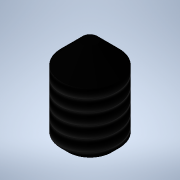
# Autodesk Inventor part: 623890036_2
Saved by Autodesk Inventor 2021 (Build 250183000, 183)
## iProperties
Created: 2026-04-17
Part Number: 623890036_2
Material: Generic
Catalog Web Link: www.3dfindit.com
Description: gst_din_4027-Grub screw, Adjusting Rings (Shaft Collars with Set Screw)  DIN 705 A
Vendor: MAEDLER
Document SubType Name: Modeling
Designer: psAdmin
Manufacturer: MAEDLER
Mass: 0.00736438 g
Surface Area: 0.231524 cm^2
Volume: 0.00736438 cm^3
Density: 1 g/cm^3
Appearance: PSOLRGB-44-44-44
Category: PARTsolutions
Company: MAEDLER
Title: 623890036
Author: Cadenas PARTsolutions
Comments: Grub screw, Adjusting Rings (Shaft Collars with Set Screw)  DIN 705 A
PSOL_IDENT_0: {$CADENAS_DATA/23d-libs/maedler/antriebselemente/klemmringe_stellringe/stellringe/din705a/din_705a_i
PSOL_IDENT_1: s_4027/gst_din_4027.prj},168 {VTYP=3D},{NB=623890036_2},{LINA=623890036},{NN=gst_din_4027},{DATE=01.
PSOL_IDENT_2: 12.2025 10:57:12},{GEOMDATE=20.02.2024 10:31:27},{VERSION=},{LINEID=2570},{WBVAR=},{WBNUMERIC=}  {NB=
PSOL_IDENT_3: 623890036_2},{LINA=623890036},{KT=DUMMY},{ARTNR=623890036},{WEBSHOP=Produktdetails / Katalogseite /
PSOL_IDENT_4: Montageanleitung},{MATK=Stahl brüniert},{MAT=Stahl brüniert, Gewindestift mit Festigkeit 45H oder 12
PSOL_IDENT_5: .9, schwarz},{AUSF=mit 1x Gewindestift mit Innensechskant DIN EN ISO 4027},{D1=3},{D2=7},{B=5},{SCHR=
PSOL_IDENT_6: M2 x 3},{GEW=0.123},{D3=1.570},{SCHRAUBE=2.0},{DD1=0.00},{N=0.0},{T=0.0},{DDD1=0.5},{SW=0.9},{T1=0.8
PSOL_IDENT_7: },{SCHRL=3},{SCHRUEB=1.0},{TYP=2},{CTN=73182900}
NB: 623890036_2
NN: gst_din_4027
NT: Grub screw, Adjusting Rings (Shaft Collars with Set Screw)  DIN 705 A
NBSYN: $ARTNR._2
LINA: 623890036
CATALOG: MÄDLER
ARTNR: 623890036
WEBSHOP: Produktdetails / Katalogseite / Montageanleitung
MATK: Stahl brüniert
MAT: Stahl brüniert, Gewindestift mit Festigkeit 45H oder 12.9, schwarz
AUSF: mit 1x Gewindestift mit Innensechskant DIN EN ISO 4027
D1: 3
D2: 7
B: 5
SCHR: M2 x 3
GEW: 0.123
D3: 1.57
SCHRAUBE: 2
DD1: 0
N: 0
T: 0
DDD1: 0.5
SW: 0.9
T1: 0.8
SCHRL: 3
SCHRUEB: 1
TYP: 2
CTN: 73182900
SUPPLIER: MAEDLER
ARTICLENO: 623890036_2
BOMINFO: 623890036
CREATOR: CADENAS GmbH
Autodesk Inventor part; units mm, degrees
sketch "Sketch_4" plane through (0, 0, 0) normal (0, 0, 1) x (1, 0, 0)
  line L0 (0, 0) -> (0, -3)
  line L1 (0, -3) -> (-0.7545, -3)
  line L2 (-0.7545, -3) -> (-1, -2.7545)
  line L3 (-1, -2.7545) -> (-1, -0.75)
  line L4 (-1, -0.75) -> (-0.25, 0)
  line L5 (-0.25, 0) -> (0, 0)
  line L6 (0, 0) -> (0, -3)
  constraints: 14 end point
revolve "Revolution1" add sketch "Sketch_4" angle 360 about axis through (0, 0, 0) along (0, 1, 0)
thread "Thread1" size "M2x0.4" class "6g" standard "ISO Metric profile" full length
sketch "Sketch_6" plane through (0, -3, 0) normal (0, 1, 0) x (1, 0, 0)
  line L0 (-0.45, -0.2598) -> (0, -0.5196)
  line L1 (0, -0.5196) -> (0.45, -0.2598)
  line L2 (0.45, -0.2598) -> (0.45, 0.2598)
  line L3 (0.45, 0.2598) -> (0, 0.5196)
  line L4 (0, 0.5196) -> (-0.45, 0.2598)
  line L5 (-0.45, 0.2598) -> (-0.45, -0.2598)
  constraints: 12 end point
extrude "Extrusion1" cut sketch "Sketch_6" along normal blind 0.8
ref_plane "gst_27434_4027_XY" through (0, -2, 0) normal (0, 1, 0) x (1, 0, 0)
ref_plane "gst_27434_4027_YZ" through (0, -2, 0) normal (1, 0, 0) x (0, 0, -1)
ref_plane "gst_27434_4027_ZX" through (0, -2, 0) normal (0, 0, -1) x (0, 1, 0)
body "Solid1"
